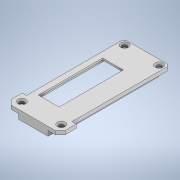
# Autodesk Inventor part: Case_top_new
Saved by Autodesk Inventor 2020 (Build 240168000, 168)
## iProperties
Created: 2022-05-01
Part Number: Case_top_new
Material: Типовые
Document SubType Name: Modeling
Designer: NoName
Density: 1 g/cm^3
Appearance: По умолчанию
Author: NoName
Autodesk Inventor part; units mm, degrees
ref_plane "YZ Plane" through (0, 0, 0) normal (1, 0, 0) x (0, 1, 0)
ref_plane "XZ Plane" through (0, 0, 0) normal (0, 1, 0) x (-1, 0, 0)
ref_plane "XY Plane" through (0, 0, 0) normal (0, 0, 1) x (1, 0, 0)
sketch "Эскиз1" plane through (0, 0, 0) normal (0, 1, 0) x (-1, 0, 0)
  line L0 (0, 0) -> (0, -46)
  line L1 (0, 0) -> (10.9, 0)
  line L2 (10.9, 0) -> (10.9, -6.5)
  line L3 (10.9, -6.5) -> (9.2, -6.5)
  line L4 (9.2, -6.5) -> (9.2, -46)
  line L5 (9.2, -46) -> (0, -46)
  line L6 (0, 0) -> (-10.9, 0)
  line L7 (-10.9, 0) -> (-10.9, -6.5)
  line L8 (-10.9, -6.5) -> (-9.2, -6.5)
  line L9 (-9.2, -6.5) -> (-9.2, -46)
  line L10 (-9.2, -46) -> (0, -46)
  dimension "d1" = 6.5
  dimension "d2" = 46
  dimension "d3" = 18.4
  dimension "d4" = 21.8
  constraints: 22 end point, 4 symmetric about line, 3 horizontal, 2 perpendicular, 1 vertical
  measures "d1" distance from line of L2.end L1
  measures "d2" distance from line of L1 L4.end
  measures "d3" distance between parallel lines of L9 L4
  measures "d4" distance between parallel lines of L7 L2
extrude "Выдавливание1" add sketch "Эскиз1" along normal blind 1.5
chamfer "Фаска1" distance 2 angle 45 2 edges at (10.9, 0.75, 0) (-10.9, 0.75, 0)
chamfer "Фаска2" distance 1 angle 45 2 edges at (9.2, 0.75, -46) (-9.2, 0.75, -46)
sketch "Эскиз2" plane through (0, 1.5, 0) normal (0, 1, 0) x (1, 0, 0)
  line L0 (0, 0) -> (0, 46)
  line L1 (8.2, 46) -> (-8.2, 46) projected
  line L2 (-8.9, 0) -> (8.9, 0) projected
  point P0 (-8, 3.4)
  point P1 (8, 3.4)
  point P2 (-7, 44)
  point P3 (7, 44)
  dimension "d20" = 3.4
  dimension "d21" = 16
  dimension "d22" = 14
  dimension "d23" = 44
  constraints: 2 end point, 2 symmetric about line, 1 midpoint
  measures "d20" distance from line of L2 point (8, 3.4)
  measures "d21" distance of point (-8, 3.4) point (8, 3.4)
  measures "d22" distance of point (7, 44) point (-7, 44)
  measures "d23" distance from line of L2 point (7, 44)
hole "Отверстие1" at (-8, 1.5, -3.4) at (8, 1.5, -3.4) at (-7, 1.5, -44) at (7, 1.5, -44) direction (0, -1, 0) diameter 2 end through all countersink diameter 3.2 countersink angle 90
sketch "Эскиз3" plane through (0, 0, 0) normal (0, -1, 0) x (1, 0, 0)
  line L0 (8.7, -6.9) -> (0, -6.9)
  line L1 (-8.9, 0) -> (8.9, 0) projected
  line L2 (8.7, -6.9) -> (8.7, -42)
  line L3 (10.9, -2) -> (10.9, -6.5) projected
  line L4 (8.7, -42) -> (6.2, -42)
  line L5 (4.2, -44) -> (4.2, -44)
  line L6 (4.2, -44) -> (0, -44)
  line L7 (8.7, -6.9) -> (5.8, -6.9)
  line L8 (0, 0) -> (0, -46)
  line L9 (8.2, -46) -> (-8.2, -46) projected
  arc A0 (6.2, -42) -> (4.2, -44) centre (6.2, -44) ccw
  line L10 (-8.7, -6.9) -> (0, -6.9)
  line L11 (-8.7, -6.9) -> (-8.7, -42)
  line L12 (-8.7, -42) -> (-6.2, -42)
  line L13 (-4.2, -44) -> (-4.2, -44)
  line L14 (-4.2, -44) -> (0, -44)
  line L15 (-8.7, -6.9) -> (-5.8, -6.9)
  arc A1 (-4.2, -44) -> (-6.2, -42) centre (-6.2, -44) ccw
  circle A2 centre (-7, -44) radius 1 projected
  circle A3 centre (-8, -3.4) radius 1 projected
  circle A4 centre (8, -3.4) radius 1 projected
  circle A5 centre (7, -44) radius 1 projected
  line L16 (-8.2, -46) -> (-9.2, -45) projected
  line L17 (8.2, -46) -> (-8.2, -46) projected
  line L18 (9.2, -45) -> (8.2, -46) projected
  line L19 (9.2, -6.5) -> (9.2, -45) projected
  line L20 (10.9, -6.5) -> (9.2, -6.5) projected
  line L21 (10.9, -2) -> (10.9, -6.5) projected
  line L22 (8.9, 0) -> (10.9, -2) projected
  line L23 (-8.9, 0) -> (8.9, 0) projected
  line L24 (-10.9, -2) -> (-8.9, 0) projected
  line L25 (-10.9, -6.5) -> (-10.9, -2) projected
  line L26 (-9.2, -6.5) -> (-10.9, -6.5) projected
  line L27 (-9.2, -45) -> (-9.2, -6.5) projected
  dimension "d24" = 6.9
  dimension "d25" = 2.2
  dimension "d26" = 42
  dimension "d27" = 44
  dimension "d28" = 6.7
  dimension "d30" = 2
  constraints: 26 end point, 7 symmetric about line, 4 point on circle, 3 point on line, 2 centre point, 2 horizontal, 2 tangent, 2 vertical, 1 midpoint, 1 perpendicular, 1 other
  measures "d24" distance between parallel lines of L1 L0
  measures "d25" distance between parallel lines of L3 L2
  measures "d26" distance between parallel lines of L1 L4
  measures "d27" distance between parallel lines of L1 L6
  measures "d28" distance between parallel lines of L3 L5
  measures "d30" radius of A0
extrude "Выдавливание2" add sketch "Эскиз3" along normal blind 0.8 contours L2 L4 A0 L6 L8 L0 | L8 L14 A1 L12 L11 L10
sketch "Эскиз5" plane through (0, -0.8, 0) normal (0, -1, 0) x (1, 0, 0)
  line L0 (-7.9, -42) -> (4.3, -42)
  line L1 (4.3, -42) -> (4.3, -8)
  line L2 (4.3, -8) -> (-7.9, -8)
  line L3 (-7.9, -8) -> (-7.9, -42)
  line L4 (-10.9, -6.5) -> (-10.9, -2) projected
  line L5 (9.2, -6.5) -> (9.2, -45) projected
  line L6 (-8.9, 0) -> (8.9, 0) projected
  line L7 (8.2, -46) -> (-8.2, -46) projected
  line L8 (-4.4, -42) -> (-4.4, -39)
  line L9 (-4.4, -39) -> (-7.9, -39)
  point P0 (0, 0)
  dimension "d33" = 3
  dimension "d35" = 8
  dimension "d36" = 4
  dimension "d40" = 31
  dimension "d41" = 3.5
  dimension "d55" = 12.2
  constraints: 12 end point, 3 perpendicular, 2 parallel, 2 point on line, 1 horizontal
  measures "d33" distance between parallel lines of L4 L3
  measures "d35" distance between parallel lines of L6 L2
  measures "d36" distance between parallel lines of L7 L0
  measures "d40" distance between parallel lines of L2 L9
  measures "d41" distance between parallel lines of L3 L8
  measures "d55" distance between parallel lines of L3 L1
extrude "Выдавливание3" cut sketch "Эскиз5" against normal blind 1.6 contours L8 L9 L3 L2 L1 L0
sketch "Эскиз6" plane through (0, 1.5, 0) normal (0, 1, 0) x (1, 0, 0)
  line L0 (-6.9, 9) -> (1.5, 9)
  line L1 (1.5, 9) -> (1.5, 35)
  line L2 (1.5, 35) -> (-6.9, 35)
  line L3 (-6.9, 35) -> (-6.9, 9)
  line L4 (-8.9, 0) -> (8.9, 0) projected
  line L5 (-9.2, 45) -> (-9.2, 6.5) projected
  line L6 (-10.9, 6.5) -> (-10.9, 2) projected
  line L7 (10.9, 2) -> (10.9, 6.5) projected
  point P0 (0, 0)
  dimension "d43" = 9
  dimension "d45" = 4
  dimension "d46" = 9.4
  dimension "d47" = 26
  constraints: 8 end point, 2 parallel, 1 horizontal, 1 perpendicular
  measures "d43" distance between parallel lines of L4 L0
  measures "d45" distance between parallel lines of L6 L3
  measures "d46" distance between parallel lines of L7 L1
  measures "d47" distance between parallel lines of L0 L2
extrude "Выдавливание4" cut sketch "Эскиз6" against normal through all
fillet "Сопряжение2" radius 2 1 edges at (-0.05, 0.8, -42)
sketch "Эскиз7" plane through (0, 0, 0) normal (0, -1, 0) x (1, 0, 0)
  line L0 (-8.9, 0) -> (8.9, 0) projected
  line L1 (8.7, -6.9) -> (-8.7, -6.9) projected
  line L2 (6, 0) -> (-6, 0)
  line L3 (-6, 0) -> (-6, -6.9)
  line L4 (-6, -6.9) -> (6, -6.9)
  line L5 (6, -6.9) -> (6, 0)
  point P0 (0, 0)
  point P1 (0, 0)
  dimension "d51" = 12
  constraints: 8 end point, 2 midpoint, 2 parallel, 2 point on line, 1 horizontal, 1 perpendicular
  measures "d51" distance between parallel lines of L3 L5
extrude "Выдавливание5" add sketch "Эскиз7" along normal blind 2
